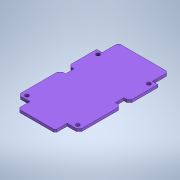
# Autodesk Inventor part: LFRboard
Saved by Autodesk Inventor 2022 (Build 260153000, 153)
## iProperties
Created: 2021-10-06
Part Number: LFRboard
Material: Generic
Document SubType Name: Modeling
Designer: Bowen O'Steen
Density: 1 g/cm^3
Appearance: Violet
Author: Bowen O'Steen
Autodesk Inventor part; units mm, degrees
ref_plane "YZ Plane" through (0, 0, 0) normal (1, 0, 0) x (0, 1, 0)
ref_plane "XZ Plane" through (0, 0, 0) normal (0, 1, 0) x (-1, 0, 0)
ref_plane "XY Plane" through (0, 0, 0) normal (0, 0, 1) x (1, 0, 0)
sketch "Sketch1" plane through (0, 0, 0) normal (0, 1, 0) x (-1, 0, 0)
  line L0 (18, 30.25) -> (-18, 30.25) construction
  line L1 (-18, 30.25) -> (-18, -32.75) construction
  line L2 (-18, -32.75) -> (18, -32.75) construction
  line L3 (18, -32.75) -> (18, 30.25) construction
  line L4 (11, 30.25) -> (-11, 30.25)
  line L5 (11, 30.25) -> (11, 23.25)
  line L6 (11, 23.25) -> (18, 23.25)
  line L7 (14.75, -32.75) -> (-14.75, -32.75)
  line L8 (14.75, -32.75) -> (14.75, -23.25)
  line L9 (14.75, -23.25) -> (18, -23.25)
  line L10 (14.75, 0) -> (18, 0)
  line L11 (-11, 30.25) -> (-11, 23.25)
  line L12 (-11, 23.25) -> (-18, 23.25)
  line L13 (-14.75, -32.75) -> (-14.75, -23.25)
  line L14 (-14.75, -23.25) -> (-18, -23.25)
  line L15 (18, 23.25) -> (18, -23.25)
  line L16 (-18, -23.25) -> (-18, 23.25)
  point P0 (0, 0)
  point P1 (0, 30.25)
  point P2 (0, -32.75)
  point P3 (-18, -6.9939)
  point P4 (18, 0)
  dimension "d0" = 36
  dimension "d1" = 63
  dimension "d2" = 22
  dimension "d3" = 7
  dimension "d4" = 29.5
  dimension "d5" = 9.5
  dimension "d10" = 7
  dimension "d11" = 9.5
  constraints: 34 end point, 7 perpendicular, 6 point on line, 5 midpoint, 4 horizontal, 2 collinear, 2 horizontal alignment, 2 parallel, 2 vertical, 1 vertical alignment
  measures "d0" distance of L0.start L0.end
  measures "d1" distance of L2.end L0.start
  measures "d2" distance of L4.start L4.end
  measures "d3" distance of L4.start L5.end
  measures "d4" distance of L7.start L7.end
  measures "d5" distance of L7.start L8.end
  measures "d10" distance between parallel lines of L0 L12
  measures "d11" distance of L7.end L13.end
extrude "Extrusion1" add sketch "Sketch1" along normal blind 1.57
chamfer "Chamfer2" distance 1 angle 45 4 edges at (11, 0.785, 30.25) (-11, 0.785, 30.25) (14.75, 0.785, -32.75) (-14.75, 0.785, -32.75)
sketch "Sketch2" plane through (0, 1.57, 0) normal (0, 1, 0) x (1, 0, 0)
  line L0 (-18, -23.25) -> (-11, -23.25) projected
  line L1 (-18, 23.25) -> (-18, -23.25) projected
  point P0 (0, 0)
  point P1 (15, -21)
  point P2 (15, 21)
  point P3 (-15, -21)
  point P4 (-15, 21)
  dimension "d20" = 42
  dimension "d21" = 42
  dimension "d22" = 30
  dimension "d28" = 2.25
  dimension "d36" = 3
  constraints: 2 vertical alignment, 1 horizontal alignment
  measures "d20" distance of point (15, 21) point (15, -21)
  measures "d21" distance of point (-15, 21) point (-15, -21)
  measures "d22" distance of point (15, -21) point (-15, -21)
  measures "d28" distance from line of L0 point (-15, -21)
  measures "d36" distance from line of L1 point (-15, -21)
hole "Hole1" at (15, 1.57, 21) at (15, 1.57, -21) at (-15, 1.57, 21) at (-15, 1.57, -21) direction (0, -1, 0) diameter 2.2 end through all clearance for "Flat Head Machine Screw" size "M2" standard "Ansi Metric M Profile"
sketch "Sketch3" plane through (0, 1.57, 0) normal (0, 1, 0) x (1, 0, 0)
  line L0 (-18, 1.5) -> (-14.75, 1.5)
  line L1 (-14.75, 1.5) -> (-14.75, 6.5)
  line L2 (-14.75, 6.5) -> (-18, 6.5)
  line L3 (-18, 23.25) -> (-18, -23.25) projected
  circle A0 centre (-15, 21) radius 1.1 projected
  line L4 (0, 0) -> (0, 8.9759) construction
  line L5 (18, 1.5) -> (14.75, 1.5)
  line L6 (14.75, 1.5) -> (14.75, 6.5)
  line L7 (14.75, 6.5) -> (18, 6.5)
  line L8 (18, 23.25) -> (18, -21.75)
  point P0 (-18, -21.75)
  point P1 (-14.75, 4)
  dimension "d37" = 5
  dimension "d38" = 3.25
  dimension "d39" = 3.25
  dimension "d40" = 17
  constraints: 16 end point, 6 symmetric about line, 2 perpendicular, 2 point on line, 1 horizontal, 1 midpoint, 1 vertical
  measures "d37" distance of L0.end L1.end
  measures "d38" distance of L0.start L0.end
  measures "d39" distance of L1.end L2.end
  measures "d40" vertical distance of A0.centre point (-14.75, 4)
extrude "Extrusion2" cut sketch "Sketch3" against normal through all contours L3 L2 L1 L0 | L5 L6 L7 L8
chamfer "Chamfer3" distance 1.5 angle 45 6 edges at (-18, 0.785, 23.25) (18, 0.785, 23.25) (18, 0.785, -1.5) (18, 0.785, -6.5) (-18, 0.785, -1.5) (-18, 0.785, -6.5)
equation "\"d21\" = d20"
equation "\"d39\" = d38"
body "Solid1"
